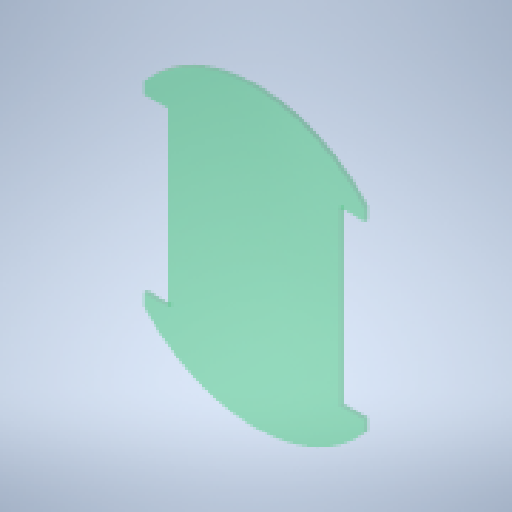
# Autodesk Inventor part: BaseBoard1
Saved by Autodesk Inventor 2025.3 (Build 293356000, 356)
## iProperties
Created: 2025-05-26
Part Number: BaseBoard1
Material: 一般
Document SubType Name: Modeling
Designer: yamashita1
Density: 1 g/cm^3
Appearance: 滑らか - 濃い深緑
Author: yamashita1
Autodesk Inventor part; units mm, degrees
ref_plane "YZ Plane" through (0, 0, 0) normal (1, 0, 0) x (0, 1, 0)
ref_plane "XZ Plane" through (0, 0, 0) normal (0, 1, 0) x (-1, 0, 0)
ref_plane "XY Plane" through (0, 0, 0) normal (0, 0, 1) x (1, 0, 0)
sketch "スケッチ1" plane through (0, 0, 0) normal (0, 0, 1) x (1, 0, 0)
  circle A0 centre (0, 0) radius 65 construction
  line L0 (-42.5, 65) -> (42.5, 65) construction
  line L1 (42.5, 65) -> (42.5, -65) construction
  line L2 (42.5, -65) -> (-42.5, -65) construction
  line L3 (-42.5, -65) -> (-42.5, 65) construction
  arc A1 (42.5, 49.1808) -> (-42.5, 49.1808) centre (0, 0) ccw
  arc A2 (-42.5, -49.1808) -> (42.5, -49.1808) centre (0, 0) ccw
  line L4 (0, 76.204) -> (0, -76.204) construction
  line L5 (-73.9944, 0) -> (73.9944, 0) construction
  line L6 (-42.5, 49.1808) -> (-42.5, -49.1808)
  line L7 (42.5, 49.1808) -> (42.5, -49.1808)
  point P0 (0, -65)
  point P1 (-42.5, 0)
  dimension "d0" = 130
  dimension "d1" = 85
  constraints: 16 end point, 9 point on circle, 4 midpoint, 3 centre point, 3 coincident, 3 parallel, 3 point on line, 2 horizontal, 2 tangent, 1 collinear, 1 concentric, 1 horizontal alignment, 1 perpendicular, 1 vertical, 1 vertical alignment
  measures "d0" diameter of A0
  measures "d1" distance of L1.end L2.end
extrude "基板" add sketch "スケッチ1" along normal blind 1.6
sketch "スケッチ2" plane through (0, 0, 1.6) normal (0, 0, 1) x (1, 0, 0)
  line L0 (-58.3969, 0) -> (58.3969, 0) construction
  line L1 (0, 57.0916) -> (0, -57.0916) construction
  line L2 (-42.5, 49.1808) -> (-42.5, -49.1808) construction
  point P0 (0, 0)
  point P1 (0, 0)
  point P2 (-36.5, 9)
  point P3 (-36.5, -9)
  point P4 (-30.5, 9)
  point P5 (-30.5, -9)
  point P6 (36.5, 9)
  point P7 (36.5, -9)
  point P8 (30.5, -9)
  point P9 (30.5, 9)
  dimension "d8" = 18
  dimension "d9" = 6
  dimension "d18" = 6
  constraints: 6 horizontal alignment, 4 end point, 3 symmetric about line, 3 vertical alignment, 2 midpoint, 1 coincident, 1 horizontal, 1 vertical
  measures "d8" distance of point (-36.5, -9) point (-36.5, 9)
  measures "d9" distance from line of L2 point (-36.5, 9)
  measures "d18" distance of point (-30.5, 9) point (-36.5, 9)
hole "ギヤボックス取付穴" at (-36.5, 9, 1.6) at (-36.5, -9, 1.6) at (-30.5, 9, 1.6) at (-30.5, -9, 1.6) at (36.5, 9, 1.6) at (36.5, -9, 1.6) at (30.5, -9, 1.6) at (30.5, 9, 1.6) direction (0, 0, -1) diameter 2.1 end through all
sketch "スケッチ3" plane through (0, 0, 1.6) normal (0, 0, 1) x (1, 0, 0)
  line L0 (-55.3039, 0) -> (55.3039, 0) construction
  line L1 (-10.5, 7.5) -> (-25.5, 7.5)
  line L2 (-25.5, 7.5) -> (-25.5, -7.5)
  line L3 (-25.5, -7.5) -> (-10.5, -7.5)
  line L4 (-10.5, -7.5) -> (-10.5, 7.5)
  line L5 (10.5, 7.5) -> (25.5, 7.5)
  line L6 (25.5, 7.5) -> (25.5, -7.5)
  line L7 (25.5, -7.5) -> (10.5, -7.5)
  line L8 (10.5, -7.5) -> (10.5, 7.5)
  line L9 (0, 63.8945) -> (0, -63.8945) construction
  circle A0 centre (-30.5, 9) radius 1.05 projected
  point P0 (0, 0)
  point P1 (0, 0)
  point P2 (-10.5, 0)
  dimension "d19" = 20
  dimension "d20" = 15
  dimension "d21" = 15
  constraints: 20 end point, 4 parallel, 3 horizontal, 3 midpoint, 3 point on line, 2 perpendicular, 1 coincident, 1 collinear, 1 vertical, 1 other
  measures "d19" distance from line of A0.centre L4
  measures "d20" distance of L3.end L1.start
  measures "d21" distance of L2.end L3.end
extrude "エンコーダ取出し穴" cut sketch "スケッチ3" against normal blind 1.6 contours L4 L3 L2 L1 | L5 L6 L7 L8
